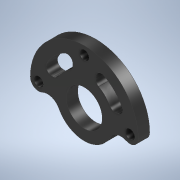
# Autodesk Inventor part: MotorSpacer
Saved by Autodesk Inventor 2020 (Build 240168000, 168)
## iProperties
Created: 2019-06-23
Part Number: MotorSpacer
Material: ABS Plastic
Document SubType Name: Modeling
Designer: Connor
Density: 1.06 g/cm^3
Appearance: Glossy - Black
Author: Connor
Autodesk Inventor part; units mm, degrees
ref_plane "YZ Plane" through (0, 0, 0) normal (1, 0, 0) x (0, 1, 0)
ref_plane "XZ Plane" through (0, 0, 0) normal (0, 1, 0) x (-1, 0, 0)
ref_plane "XY Plane" through (0, 0, 0) normal (0, 0, 1) x (1, 0, 0)
sketch "Sketch1" plane through (0, 0, 0) normal (0, 0, 1) x (1, 0, 0)
  circle A0 centre (0, 0) radius 10
  circle A1 centre (0, 25.4) radius 2.6035
  circle A2 centre (25.4, 0) radius 2.6035
  circle A3 centre (0, 0) radius 25.4 construction
  circle A4 centre (0, 0) radius 30
  circle A5 centre (0, 25.4) radius 4.6
  circle A6 centre (25.4, 0) radius 4.6
  circle A7 centre (0, 0) radius 15.875
  circle A8 centre (-25.4, 0) radius 2.6035
  circle A9 centre (0, -25.4) radius 2.6035
  circle A10 centre (-25.4, 0) radius 4.6
  circle A11 centre (0, -25.4) radius 4.6
  circle A12 centre (-20.3794, -10.5265) radius 7.0625
  circle A13 centre (20.3794, -10.5265) radius 7.0625
  point P0 (30, 0)
  point P1 (0, 30)
  point P2 (14.1046, -7.2854)
  point P3 (23.4198, -4.1519)
  point P4 (-30, 0)
  point P5 (-23.4198, -4.1519)
  point P6 (-14.1046, -7.2854)
  dimension "d2" = 50.8
  dimension "d3" = 20
  dimension "d6" = 5.207
  dimension "d7" = 60
  dimension "d8" = 31.75
  constraints: 14 centre point, 10 tangent, 8 coincident, 4 point on circle, 3 equal radius, 2 horizontal alignment, 2 vertical alignment
  measures "d2" diameter of A3
  measures "d3" diameter of A0
  measures "d6" diameter of A1
  measures "d7" diameter of A4
  measures "d8" diameter of A7
extrude "Extrusion1" add sketch "Sketch1" along normal blind 6.35 contours A5 | A6 A13 A7 A12 A10 A4 | A6 | A10 | A7
sketch "Sketch2" plane through (0, 0, 6.35) normal (0, 0, 1) x (1, 0, 0)
  circle A0 centre (0, 0) radius 10 construction
  arc A1 (30, 0) -> (-30, 0) centre (0, 0) ccw construction
  line L0 (0, 0) -> (0, 30) construction
  arc A2 (-11.002, 20.9351) -> (-20.9351, 11.002) centre (0, 0) ccw
  arc A3 (-7.9761, 14.2725) -> (-14.2725, 7.9761) centre (0, 0) ccw
  line L1 (-6.35, 18.1246) -> (-6.35, 17.0441)
  line L2 (-17.0441, 6.35) -> (-18.1246, 6.35)
  arc A4 (-20.9351, 11.002) -> (-18.1246, 6.35) centre (-18.1246, 9.525) ccw
  arc A5 (-17.0441, 6.35) -> (-14.2725, 7.9761) centre (-17.0441, 9.525) ccw
  arc A6 (-7.9761, 14.2725) -> (-6.35, 17.0441) centre (-9.525, 17.0441) ccw
  arc A7 (-6.35, 18.1246) -> (-11.002, 20.9351) centre (-9.525, 18.1246) ccw
  arc A8 (20.9351, 11.002) -> (11.002, 20.9351) centre (0, 0) ccw
  arc A9 (14.2725, 7.9761) -> (7.9761, 14.2725) centre (0, 0) ccw
  line L3 (6.35, 18.1246) -> (6.35, 17.0441)
  line L4 (17.0441, 6.35) -> (18.1246, 6.35)
  arc A10 (18.1246, 6.35) -> (20.9351, 11.002) centre (18.1246, 9.525) ccw
  arc A11 (14.2725, 7.9761) -> (17.0441, 6.35) centre (17.0441, 9.525) ccw
  arc A12 (6.35, 17.0441) -> (7.9761, 14.2725) centre (9.525, 17.0441) ccw
  arc A13 (11.002, 20.9351) -> (6.35, 18.1246) centre (9.525, 18.1246) ccw
  point P0 (-6.35, 22.7816)
  point P1 (-22.7816, 6.35)
  point P2 (-6.35, 15.0665)
  point P3 (-15.0665, 6.35)
  dimension "d9" = 6.35
  dimension "d10" = 6.35
  dimension "d11" = 6.35
  dimension "d12" = 6.35
  dimension "d13" = 3.175
  constraints: 29 point on circle, 12 centre point, 12 symmetric about line, 10 end point, 8 tangent, 4 point on line, 3 coincident, 3 equal radius, 2 vertical, 1 horizontal, 6 other
  measures "d9" radial gap between concentric circles of A2 A1
  measures "d10" radial gap between concentric circles of A0 A3
  measures "d11" distance from line of point (0, 0) L2
  measures "d12" distance between parallel lines of L1 L0
  measures "d13" radius of A4
extrude "Extrusion2" cut sketch "Sketch2" against normal through all
equation "\"d10\" = d9"
equation "\"d11\" = d9"
equation "\"d12\" = d9"
body "Solid1"
